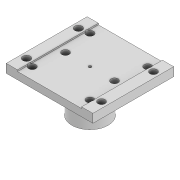
# Autodesk Inventor part: 200205 - Holder for MEMS on halfinch mount
Saved by Autodesk Inventor 2020.3 (Build 243373000, 373)
## iProperties
Created: 2019-06-07
Part Number: 200205 - Holder for MEMS on halfinch mount
Material: Generic
Document SubType Name: Modeling
Designer: kpb10108
Density: 1 g/cm^3
Appearance: Default
Author: kpb10108
Autodesk Inventor part; units mm, degrees
ref_plane "YZ Plane" through (0, 0, 0) normal (1, 0, 0) x (0, 1, 0)
ref_plane "XZ Plane" through (0, 0, 0) normal (0, 1, 0) x (-1, 0, 0)
ref_plane "XY Plane" through (0, 0, 0) normal (0, 0, 1) x (1, 0, 0)
sketch "Sketch1" plane through (0, 0, 0) normal (0, 1, 0) x (-1, 0, 0)
  circle A0 centre (0, 0) radius 6.25
  dimension "d0" = 12.5
  constraints: 1 centre point, 1 coincident
  measures "d0" diameter of A0
extrude "Extrusion1" add sketch "Sketch1" along normal blind 12
sketch "Sketch2" plane through (0, 12, 0) normal (0, 1, 0) x (1, 0, 0)
  line L0 (-15, 14) -> (15, 14)
  line L1 (15, 14) -> (15, -14)
  line L2 (15, -14) -> (-15, -14)
  line L3 (-15, -14) -> (-15, 14)
  point P0 (0, 0)
  dimension "d3" = 30
  dimension "d4" = 28
  dimension "d5" = 14
  dimension "d6" = 15
  constraints: 8 end point, 2 parallel, 1 horizontal, 1 perpendicular
  measures "d3" distance of L0.start L0.end
  measures "d4" distance of L0.end L1.end
  measures "d5" distance from line of point (0, 0) L0
  measures "d6" distance from line of L1 point (0, 0)
extrude "Extrusion2" add sketch "Sketch2" along normal blind 3
sketch "Sketch3" plane through (0, 15, 0) normal (0, 1, 0) x (1, 0, 0)
  line L0 (-15, -14) -> (15, -14) projected
  line L1 (15, 14) -> (-15, 14) projected
  line L2 (11.1, -14) -> (-11.1, -14)
  line L3 (-11.1, -14) -> (-11.1, 14)
  line L4 (-11.1, 14) -> (11.1, 14)
  line L5 (11.1, 14) -> (11.1, -14)
  line L6 (-15, 14) -> (-15, -14) projected
  point P0 (0, 0)
  point P1 (11.1, 14)
  point P2 (-11.1, -14)
  dimension "d9" = 22.2
  dimension "d10" = 3.9
  constraints: 8 end point, 2 parallel, 2 point on line, 1 horizontal, 1 perpendicular
  measures "d9" distance between parallel lines of L3 L5
  measures "d10" distance between parallel lines of L6 L3
extrude "Extrusion3" cut sketch "Sketch3" against normal blind 0.5 contours L3 L1 L5 L0
sketch "Sketch4" plane through (0, 14.5, 0) normal (0, 1, 0) x (1, 0, 0)
  circle A0 centre (8.5, 0) radius 1.25
  circle A1 centre (-8.5, 0) radius 1.25
  point P0 (0, 0)
  dimension "d13" = 2.5
  dimension "d14" = 8.5
  dimension "d15" = 2.5
  dimension "d16" = 8.5
  constraints: 2 centre point
  measures "d13" diameter of A0
  measures "d14" distance of A0.centre point (0, 0)
  measures "d15" diameter of A1
  measures "d16" distance of A1.centre point (0, 0)
extrude "Extrusion4" cut sketch "Sketch4" against normal blind 5
sketch "Sketch5" plane through (0, 12, 0) normal (0, -1, 0) x (1, 0, 0)
  line L0 (7.4961, 2.1) -> (15, 2.1)
  line L1 (15, 2.1) -> (15, -2.1)
  line L2 (15, -2.1) -> (7.4961, -2.1)
  line L3 (7.4961, -2.1) -> (7.4961, 2.1)
  line L4 (15, 14) -> (15, -14) projected
  circle A0 centre (8.5, 0) radius 1.25 projected
  line L5 (9.75, 2.1) -> (10.9437, -0.0325)
  line L6 (10.9437, -0.0325) -> (9.6937, -2.1325)
  line L7 (9.6937, -2.1325) -> (7.25, -2.1)
  line L8 (7.25, -2.1) -> (6.0563, 0.0325)
  line L9 (6.0563, 0.0325) -> (7.3063, 2.1325)
  line L10 (7.3063, 2.1325) -> (9.75, 2.1)
  line L11 (-15, -14) -> (-15, 14) projected
  line L12 (-15, -2.1) -> (-7.25, -2.1)
  line L13 (-7.25, -2.1) -> (-7.25, 2.1)
  line L14 (-7.25, 2.1) -> (-15, 2.1)
  line L15 (-15, 2.1) -> (-15, -2.1)
  circle A1 centre (-8.5, 0) radius 1.25 projected
  line L16 (-7.25, 2.1) -> (-6.0563, -0.0325)
  line L17 (-6.0563, -0.0325) -> (-7.3063, -2.1325)
  line L18 (-7.3063, -2.1325) -> (-9.75, -2.1)
  line L19 (-9.75, -2.1) -> (-10.9437, 0.0325)
  line L20 (-10.9437, 0.0325) -> (-9.6937, 2.1325)
  line L21 (-9.6937, 2.1325) -> (-7.25, 2.1)
  point P0 (0, 0)
  point P1 (9.713, -2.1)
  point P2 (-9.713, 2.1)
  dimension "d19" = 4.2
  dimension "d20" = 0
  dimension "d21" = 2.1
  dimension "d24" = 4.2
  dimension "d25" = 2.1
  constraints: 40 end point, 4 parallel, 2 coincident, 2 horizontal, 2 perpendicular, 2 point on line, 26 other
  measures "d19" distance of L0.end L1.end
  measures "d20" distance between parallel lines of L4 L1
  measures "d21" distance from line of point (0, 0) L0
  measures "d24" distance of L13.end L12.end
  measures "d25" distance from line of point (0, 0) L12
extrude "Extrusion5" cut sketch "Sketch5" along normal blind 3 contours L3 A0 L2 L6 L7 L8 L9 L10 L0 | L0 L5 L6 L2 L3 A0 | L0 L1 L2 L6 L5 | A0 L3 | L3 A0 | L11 L14 L20 L19 L12 | A1 | L19 L20 L14 L13 L17 L12 | L12 L17 L18 | L20 L21 L14 | L16 L17 L13
sketch "Sketch6" plane through (0, 14.5, 0) normal (0, 1, 0) x (1, 0, 0)
  line L0 (-11.1, -14) -> (-11.1, 14) projected
  line L1 (-11.1, 11) -> (11.1, 11)
  line L2 (11.1, 11) -> (11.1, -11)
  line L3 (11.1, -11) -> (-11.1, -11)
  line L4 (-11.1, -11) -> (-11.1, 11)
  line L5 (-11.1, 14) -> (11.1, 14) projected
  circle A0 centre (-13, -9) radius 1.3
  line L6 (-15, -14) -> (-11.1, -14) projected
  circle A1 centre (-13, 9) radius 1.3
  line L7 (-11.1, 14) -> (-15, 14) projected
  circle A2 centre (13, 9) radius 1.25
  line L8 (11.1, 14) -> (11.1, -14) projected
  circle A3 centre (13, -9) radius 1.25
  line L9 (11.1, -14) -> (15, -14) projected
  point P0 (0, 0)
  dimension "d26" = 22.2
  dimension "d27" = 22
  dimension "d28" = 3
  dimension "d29" = 2.6
  dimension "d30" = 1.9
  dimension "d31" = 5
  dimension "d32" = 2.6
  dimension "d33" = 1.9
  dimension "d34" = 5
  dimension "d35" = 2.5
  dimension "d36" = 1.9
  dimension "d37" = 5
  dimension "d38" = 2.5
  dimension "d39" = 1.9
  dimension "d40" = 5
  constraints: 8 end point, 4 centre point, 2 parallel, 1 horizontal, 1 perpendicular, 1 point on line
  measures "d26" distance of L2.end L3.end
  measures "d27" distance of L1.end L2.end
  measures "d28" distance between parallel lines of L5 L1
  measures "d29" diameter of A0
  measures "d30" distance from line of L0 A0.centre
  measures "d31" distance from line of A0.centre L6
  measures "d32" diameter of A1
  measures "d33" distance from line of L0 A1.centre
  measures "d34" distance from line of L7 A1.centre
  measures "d35" diameter of A2
  measures "d36" distance from line of L8 A2.centre
  measures "d37" distance from line of L5 A2.centre
  measures "d38" diameter of A3
  measures "d39" distance from line of L2 A3.centre
  measures "d40" distance from line of L9 A3.centre
extrude "Extrusion6" cut sketch "Sketch6" along normal mid plane 5 contours A0 | A1 | A2 | A3
sketch "Sketch7" plane through (0, 14.5, 0) normal (0, 1, 0) x (1, 0, 0)
  circle A0 centre (-10, 10) radius 1.25
  line L0 (0, 0) -> (4.1718, 0)
  line L1 (0, 0) -> (0, 4.2645)
  circle A1 centre (10, 10) radius 1.25
  circle A2 centre (-10, -10) radius 1.25
  circle A3 centre (10, -10) radius 1.25
  dimension "d43" = 2.5
  dimension "d44" = 10
  dimension "d45" = 10
  dimension "d48" = 20
  dimension "d51" = 20
  constraints: 4 centre point, 4 end point, 2 horizontal, 2 vertical, 6 other
  measures "d43" diameter of A0
  measures "d44" horizontal distance of A0.centre L0.start
  measures "d45" horizontal distance of A0.centre L0.start
  measures "d48" distance of A0.centre A1.centre
  measures "d51" distance of A0.centre A2.centre
extrude "Extrusion7" cut sketch "Sketch7" along normal blind 10 and the other way blind 5
sketch "Sketch8" plane through (0, 12, 0) normal (0, -1, 0) x (1, 0, 0)
  arc A0 (11.1, -9.4063) -> (11.1, -10.5937) centre (10, -10) ccw projected
  circle A1 centre (10, -10) radius 2.5
  circle A2 centre (-10, -10) radius 1.25 projected
  circle A3 centre (-10, -10) radius 2.5
  arc A4 (-11.1, 9.4063) -> (-11.1, 10.5937) centre (-10, 10) ccw projected
  circle A5 centre (-10, 10) radius 2.5
  arc A6 (11.1, 10.5937) -> (11.1, 9.4063) centre (10, 10) ccw projected
  circle A7 centre (10, 10) radius 2.5
  point P0 (0, 0)
  dimension "d58" = 5
  dimension "d59" = 5
  dimension "d60" = 5
  dimension "d61" = 5
  constraints: 4 centre point, 4 coincident
  measures "d58" diameter of A1
  measures "d59" diameter of A3
  measures "d60" diameter of A5
  measures "d61" diameter of A7
extrude "Extrusion8" cut sketch "Sketch8" along normal blind 5
sketch "Sketch9" plane through (0, 14.5, 0) normal (0, 1, 0) x (1, 0, 0)
  point P0 (0, 0)
  point P1 (0, 0)
  constraints: 1 coincident
hole "Hole1" at (0, 14.5, 0) direction (0, -1, 0) diameter 1 end through all
body "Solid1"
